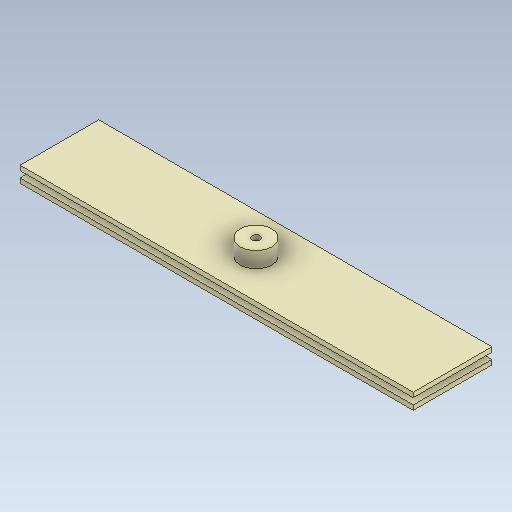
# Autodesk Inventor part: trail 7
Saved by Autodesk Inventor 2020.2 (Build 242310000, 310)
## iProperties
Created: 2020-02-14
Part Number: trail 7
Material: Polypropylene
Document SubType Name: Modeling
Designer: lenovo
Density: 0.899 g/cm^3
Appearance: Smooth - Ash
Author: lenovo
Autodesk Inventor part; units mm, degrees
ref_plane "YZ Plane" through (0, 0, 0) normal (1, 0, 0) x (0, 1, 0)
ref_plane "XZ Plane" through (0, 0, 0) normal (0, 1, 0) x (-1, 0, 0)
ref_plane "XY Plane" through (0, 0, 0) normal (0, 0, 1) x (1, 0, 0)
sketch "Sketch1" plane through (0, 0, 0) normal (0, 1, 0) x (-1, 0, 0)
  line L0 (-125, -25) -> (125, -25)
  line L1 (125, -25) -> (125, 25)
  line L2 (125, 25) -> (-125, 25)
  line L3 (-125, 25) -> (-125, -25)
  line L4 (-125, -25) -> (125, 25) construction
  line L5 (125, -25) -> (-125, 25) construction
  point P0 (0, 0)
  dimension "d0" = 250
  dimension "d1" = 50
  constraints: 12 end point, 2 midpoint, 2 parallel, 1 horizontal, 1 perpendicular
  measures "d0" distance of L2.end L1.end
  measures "d1" distance of L1.end L0.end
extrude "Extrusion1" add sketch "Sketch1" along normal blind 3
sketch "Sketch2" plane through (0, 3, 0) normal (0, 1, 0) x (1, 0, 0)
  line L0 (120, 20) -> (-120, 20)
  line L1 (-120, 20) -> (-120, -20)
  line L2 (-120, -20) -> (120, -20)
  line L3 (120, -20) -> (120, 20)
  line L4 (120, 20) -> (-120, -20) construction
  line L5 (-120, 20) -> (120, -20) construction
  point P0 (0, 0)
  dimension "d4" = 240
  dimension "d5" = 40
  constraints: 12 end point, 2 midpoint, 2 parallel, 1 horizontal, 1 perpendicular
  measures "d4" distance of L2.end L1.end
  measures "d5" distance of L1.end L0.end
extrude "Extrusion2" add sketch "Sketch2" along normal blind 4
sketch "Sketch3" plane through (0, 7, 0) normal (0, 1, 0) x (1, 0, 0)
  line L0 (125, 25) -> (-125, 25)
  line L1 (-125, 25) -> (-125, -25)
  line L2 (-125, -25) -> (125, -25)
  line L3 (125, -25) -> (125, 25)
  line L4 (125, 25) -> (-125, -25) construction
  line L5 (-125, 25) -> (125, -25) construction
  point P0 (0, 0)
  constraints: 12 end point, 2 midpoint, 2 parallel, 1 horizontal, 1 perpendicular
extrude "Extrusion3" add sketch "Sketch3" along normal blind 3
sketch "Sketch4" plane through (0, 10, 0) normal (0, 1, 0) x (1, 0, 0)
  circle A0 centre (0, 0) radius 10
  dimension "d10" = 20
  constraints: 1 centre point, 1 coincident
  measures "d10" diameter of A0
extrude "Extrusion4" add sketch "Sketch4" along normal blind 10
sketch "Sketch5" plane through (0, 20, 0) normal (0, 1, 0) x (1, 0, 0)
  circle A0 centre (0, 0) radius 2.5
  dimension "d13" = 5
  constraints: 1 centre point, 1 coincident
  measures "d13" diameter of A0
extrude "Extrusion5" cut sketch "Sketch5" against normal blind 30
body "Solid1"
